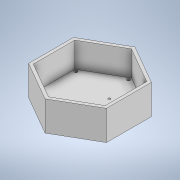
# Autodesk Inventor part: Improved Internal Base
Saved by Autodesk Inventor 2020 (Build 240168000, 168)
## iProperties
Created: 2020-02-13
Part Number: Improved Internal Base
Material: Generic
Document SubType Name: Modeling
Designer: danie
Density: 1 g/cm^3
Appearance: Default
Author: danie
Autodesk Inventor part; units mm, degrees
ref_plane "YZ Plane" through (0, 0, 0) normal (1, 0, 0) x (0, 1, 0)
ref_plane "XZ Plane" through (0, 0, 0) normal (0, 1, 0) x (-1, 0, 0)
ref_plane "XY Plane" through (0, 0, 0) normal (0, 0, 1) x (1, 0, 0)
sketch "Sketch1" plane through (0, 0, 0) normal (0, 1, 0) x (-1, 0, 0)
  line L0 (0, 0) -> (0, -70)
  line L1 (0, -70) -> (60.6218, -105)
  line L2 (60.6218, -105) -> (121.2436, -70)
  line L3 (121.2436, -70) -> (121.2436, 0)
  line L4 (121.2436, 0) -> (60.6218, 35)
  line L5 (60.6218, 35) -> (0, 0)
  line L6 (-5, 2.8868) -> (-5, -72.8868)
  line L7 (-5, -72.8868) -> (60.6218, -110.7735)
  line L8 (60.6218, -110.7735) -> (126.2436, -72.8868)
  line L9 (126.2436, -72.8868) -> (126.2436, 2.8868)
  line L10 (126.2436, 2.8868) -> (60.6218, 40.7735)
  line L11 (60.6218, 40.7735) -> (-5, 2.8868)
  line L12 (0, 0) -> (-5, 0) construction
  line L13 (-5, 2.8868) -> (0, 0) construction
  dimension "wall" = 70
  dimension "d1" = 70
  dimension "d2" = 70
  dimension "d3" = 70
  dimension "d4" = 70
  dimension "d5" = 70
  dimension "d6" = 120
  dimension "d7" = 120
  dimension "d9" = 120
  dimension "d10" = 120
  dimension "d11" = 120
  dimension "wallThickness" = 5
  dimension "d15" = 5
  dimension "d16" = 131.2436
  constraints: 28 end point, 5 equal length, 2 vertical, 1 parallel, 1 perpendicular, 1 point on line
  measures "wall" distance of L0.start L0.end
  measures "d1" distance of L0.end L1.end
  measures "d2" distance of L1.end L2.end
  measures "d3" distance of L2.end L3.end
  measures "d4" distance of L3.end L4.end
  measures "d5" distance of L0.start L4.end
  measures "d6" angle of L0 L1
  measures "d7" angle of L1 L2
  measures "d9" angle of L2 L3
  measures "d10" angle of L6 L7
  measures "d11" angle of L7 L8
  measures "wallThickness" distance between parallel lines of L6 L0
  measures "d15" distance between parallel lines of L11 L5
  measures "d16" horizontal distance of L6.start L8.end
extrude "Extrusion1" add sketch "Sketch1" along normal blind 7.5 contours L5 L4 L3 L2 L1 L0
extrude "Extrusion2" add sketch "Sketch1" along normal blind 50
sketch "Sketch2" plane through (0, 7.5, 0) normal (0, 1, 0) x (1, 0, 0)
  circle A0 centre (-4.45, 55.955) radius 1.905
  circle A1 centre (-4.45, 14.045) radius 1.905
  line L0 (-4.45, 55.955) -> (-4.45, 14.045) construction
  line L1 (0, 70) -> (0, 0) construction
  line L2 (-4.45, 14.045) -> (-48.935, 14.045) construction
  circle A2 centre (-48.935, 14.045) radius 1.905
  circle A3 centre (-48.935, 55.955) radius 1.905
  line L3 (0, 70) -> (-60.6218, 105) projected
  line L4 (0, 70) -> (-1, 70) construction
  dimension "holderRadius" = 3.81
  dimension "d22" = 3.81
  dimension "d23" = 41.91
  dimension "d24" = 4.45
  dimension "d25" = 44.485
  dimension "d26" = 3.81
  dimension "d27" = 3.81
  dimension "d28" = 41.91
  dimension "d29" = 44.485
  dimension "d30" = 1
  dimension "d31" = 14.045
  constraints: 6 end point, 4 centre point, 2 coincident, 1 horizontal, 1 perpendicular, 1 vertical
  measures "holderRadius" diameter of A0
  measures "d22" diameter of A1
  measures "d23" distance of L0.start L0.end
  measures "d24" distance from line of L1 L0.start
  measures "d25" distance of L0.end L2.end
  measures "d26" diameter of A2
  measures "d27" diameter of A3
  measures "d28" distance of L2.end A3.centre
  measures "d29" distance of L0.start A3.centre
  measures "d30" distance of L1.start L4.end
  measures "d31" distance from line of L0.start L4
extrude "Extrusion3" cut sketch "Sketch2" against normal blind 5
sketch "Sketch3" plane through (0, 7.5, 0) normal (0, 1, 0) x (1, 0, 0)
  circle A0 centre (-4.3301, 2.5) radius 2.5
  line L0 (0, 0) -> (0, 70) projected
  line L1 (0, 0) -> (-4.3301, 2.5) construction
  line L2 (0, 0) -> (5, 0) construction
  line L3 (-60.6218, -35) -> (-121.2436, 0) construction
  line L4 (-60.6218, -35) -> (-60.6218, -30) construction
  line L5 (-60.6218, -35) -> (-55.6218, -35) construction
  line L6 (-121.2436, 70) -> (-121.2436, 0) construction
  line L7 (-121.2436, 0) -> (-116.9134, 2.5) construction
  line L8 (-121.2436, 0) -> (-116.2436, 0) construction
  line L9 (-60.6218, 105) -> (-60.6218, 100) construction
  line L10 (0, 70) -> (-4.3301, 67.5) construction
  circle A1 centre (-4.3301, 67.5) radius 2.5
  line L11 (-121.2436, 70) -> (-60.6218, 105) construction
  circle A2 centre (-116.9134, 2.5) radius 2.5
  line L12 (-121.2436, 70) -> (-116.9134, 67.5) construction
  circle A3 centre (-116.9134, 67.5) radius 2.5
  circle A4 centre (-60.6218, 100) radius 2.5
  circle A5 centre (-60.6218, -30) radius 2.5
  circle A6 centre (-60.6218, -30) radius 1.25
  circle A7 centre (-116.9134, 2.5) radius 1.25
  circle A8 centre (-116.9134, 67.5) radius 1.25
  circle A9 centre (-60.6218, 100) radius 1.25
  circle A10 centre (-4.3301, 67.5) radius 1.25
  circle A11 centre (-4.3301, 2.5) radius 1.25
  dimension "holeRad" = 5
  dimension "d35" = 5
  dimension "d36" = 150
  dimension "d37" = 5
  dimension "d38" = 90
  dimension "d39" = 5
  dimension "d40" = 30
  dimension "d42" = 5
  dimension "d43" = 5
  dimension "d44" = 5
  dimension "d45" = 60
  dimension "d47" = 5
  dimension "d48" = 5
  dimension "d49" = 60
  dimension "d50" = 5
  dimension "d51" = 5
  dimension "d52" = 5
  dimension "d53" = 2.5
  dimension "d54" = 2.5
  dimension "d55" = 2.5
  dimension "d56" = 2.5
  dimension "d57" = 2.5
  dimension "d58" = 2.5
  constraints: 18 end point, 15 coincident, 12 centre point, 3 equal length, 3 horizontal, 2 vertical
  measures "holeRad" diameter of A0
  measures "d35" distance of L1.start L1.end
  measures "d36" angle of L2 L1
  measures "d37" distance of L3.start L4.end
  measures "d38" angle of L5 L4
  measures "d39" distance of L3.end L7.end
  measures "d40" angle of L8 L7
  measures "d42" distance of L9.start L9.end
  measures "d43" distance of L0.end L10.end
  measures "d44" diameter of A1
  measures "d45" angle of L0 L10
  measures "d47" diameter of A2
  measures "d48" distance of L6.start L12.end
  measures "d49" angle of L11 L12
  measures "d50" diameter of A3
  measures "d51" diameter of A4
  measures "d52" diameter of A5
  measures "d53" diameter of A6
  measures "d54" diameter of A7
  measures "d55" diameter of A8
  measures "d56" diameter of A9
  measures "d57" diameter of A10
  measures "d58" diameter of A11
extrude "Extrusion4" cut sketch "Sketch3" against normal blind 3.75
extrude "Extrusion5" cut sketch "Sketch3" against normal blind 7.5 contours A6 | A7 | A8 | A9 | A10 | A11
equation "\"d1\" = wall"
equation "\"d2\" = wall"
equation "\"d3\" = wall"
equation "\"d4\" = wall"
equation "\"d5\" = wall"
body "Solid1"
